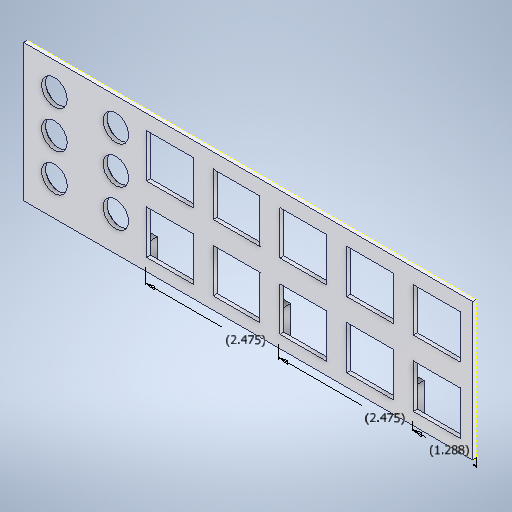
# Autodesk Inventor part: front_panel
Saved by Autodesk Inventor 2025 (Build 290162000, 162)
## iProperties
Created: 2025-05-12
Part Number: front_panel
Material: Generic
Document SubType Name: Modeling
Designer: ethan
Density: 1 g/cm^3
Appearance: PTFE
Author: ethan
Autodesk Inventor part; units mm, degrees
ref_plane "YZ Plane" through (0, 0, 0) normal (1, 0, 0) x (0, 1, 0)
ref_plane "XZ Plane" through (0, 0, 0) normal (0, 1, 0) x (-1, 0, 0)
ref_plane "XY Plane" through (0, 0, 0) normal (0, 0, 1) x (1, 0, 0)
sketch "Sketch1" plane through (0, 0, 0) normal (0, 0, 1) x (1, 0, 0)
  line L0 (0, 0) -> (-6.35, 0) construction
  line L1 (-6.35, 0) -> (-6.35, 6.35) construction
  line L2 (-6.35, 6.35) -> (0, 6.35) construction
  line L3 (0, 6.35) -> (0, 0) construction
  line L4 (-6.35, 6.35) -> (-30.1625, 6.35)
  line L5 (-30.1625, 6.35) -> (-30.1625, 28.575)
  line L6 (-30.1625, 28.575) -> (-6.35, 28.575)
  line L7 (-6.35, 28.575) -> (-6.35, 6.35)
  line L8 (-30.1625, 6.35) -> (-35.2425, 6.35) construction
  line L9 (-35.2425, 6.35) -> (-35.2425, 0) construction
  line L10 (-35.2425, 0) -> (-30.1625, 0) construction
  line L11 (-30.1625, 0) -> (-30.1625, 6.35) construction
  line L12 (-40.3225, 6.35) -> (-64.135, 6.35)
  line L13 (-64.135, 6.35) -> (-64.135, 28.575)
  line L14 (-64.135, 28.575) -> (-40.3225, 28.575)
  line L15 (-40.3225, 28.575) -> (-40.3225, 6.35)
  line L16 (-64.135, 6.35) -> (-69.215, 6.35) construction
  line L17 (-69.215, 6.35) -> (-69.215, 0) construction
  line L18 (-69.215, 0) -> (-64.135, 0) construction
  line L19 (-64.135, 0) -> (-64.135, 6.35) construction
  line L20 (-74.295, 6.35) -> (-98.1075, 6.35)
  line L21 (-98.1075, 6.35) -> (-98.1075, 28.575)
  line L22 (-98.1075, 28.575) -> (-74.295, 28.575)
  line L23 (-74.295, 28.575) -> (-74.295, 6.35)
  line L24 (-98.1075, 6.35) -> (-103.1875, 6.35) construction
  line L25 (-103.1875, 6.35) -> (-103.1875, 0) construction
  line L26 (-103.1875, 0) -> (-98.1075, 0) construction
  line L27 (-98.1075, 0) -> (-98.1075, 6.35) construction
  line L28 (-108.2675, 6.35) -> (-132.08, 6.35)
  line L29 (-132.08, 6.35) -> (-132.08, 28.575)
  line L30 (-132.08, 28.575) -> (-108.2675, 28.575)
  line L31 (-108.2675, 28.575) -> (-108.2675, 6.35)
  line L32 (-132.08, 6.35) -> (-137.16, 6.35) construction
  line L33 (-137.16, 6.35) -> (-137.16, 0) construction
  line L34 (-137.16, 0) -> (-132.08, 0) construction
  line L35 (-132.08, 0) -> (-132.08, 6.35) construction
  line L36 (-6.35, 40.005) -> (-30.1625, 40.005)
  line L37 (-30.1625, 40.005) -> (-30.1625, 62.23)
  line L38 (-30.1625, 62.23) -> (-6.35, 62.23)
  line L39 (-6.35, 62.23) -> (-6.35, 40.005)
  line L40 (-30.1625, 40.005) -> (-35.2425, 40.005) construction
  line L41 (-35.2425, 40.005) -> (-35.2425, 33.655) construction
  line L42 (-35.2425, 33.655) -> (-30.1625, 33.655) construction
  line L43 (-30.1625, 33.655) -> (-30.1625, 40.005) construction
  line L44 (-40.3225, 40.005) -> (-64.135, 40.005)
  line L45 (-64.135, 40.005) -> (-64.135, 62.23)
  line L46 (-64.135, 62.23) -> (-40.3225, 62.23)
  line L47 (-40.3225, 62.23) -> (-40.3225, 40.005)
  line L48 (-64.135, 40.005) -> (-69.215, 40.005) construction
  line L49 (-69.215, 40.005) -> (-69.215, 33.655) construction
  line L50 (-69.215, 33.655) -> (-64.135, 33.655) construction
  line L51 (-64.135, 33.655) -> (-64.135, 40.005) construction
  line L52 (-74.295, 40.005) -> (-98.1075, 40.005)
  line L53 (-98.1075, 40.005) -> (-98.1075, 62.23)
  line L54 (-98.1075, 62.23) -> (-74.295, 62.23)
  line L55 (-74.295, 62.23) -> (-74.295, 40.005)
  line L56 (-98.1075, 40.005) -> (-103.1875, 40.005) construction
  line L57 (-103.1875, 40.005) -> (-103.1875, 33.655) construction
  line L58 (-103.1875, 33.655) -> (-98.1075, 33.655) construction
  line L59 (-98.1075, 33.655) -> (-98.1075, 40.005) construction
  line L60 (-108.2675, 40.005) -> (-132.08, 40.005)
  line L61 (-132.08, 40.005) -> (-132.08, 62.23)
  line L62 (-132.08, 62.23) -> (-108.2675, 62.23)
  line L63 (-108.2675, 62.23) -> (-108.2675, 40.005)
  line L64 (-132.08, 40.005) -> (-137.16, 40.005) construction
  line L65 (-137.16, 40.005) -> (-137.16, 33.655) construction
  line L66 (-137.16, 33.655) -> (-132.08, 33.655) construction
  line L67 (-132.08, 33.655) -> (-132.08, 40.005) construction
  line L68 (0, -0.5542) -> (0, 69.2958)
  line L69 (0, 62.9458) -> (0, 69.2958)
  line L70 (-142.24, 6.35) -> (-166.0525, 6.35)
  line L71 (-166.0525, 6.35) -> (-166.0525, 28.575)
  line L72 (-166.0525, 28.575) -> (-142.24, 28.575)
  line L73 (-142.24, 28.575) -> (-142.24, 6.35)
  line L74 (-166.0525, 6.35) -> (-171.1325, 6.35) construction
  line L75 (-171.1325, 6.35) -> (-171.1325, 0) construction
  line L76 (-171.1325, 0) -> (-166.0525, 0) construction
  line L77 (-166.0525, 0) -> (-166.0525, 6.35) construction
  line L78 (-142.24, 40.005) -> (-166.0525, 40.005)
  line L79 (-166.0525, 40.005) -> (-166.0525, 62.23)
  line L80 (-166.0525, 62.23) -> (-142.24, 62.23)
  line L81 (-142.24, 62.23) -> (-142.24, 40.005)
  line L82 (-166.0525, 40.005) -> (-171.1325, 40.005) construction
  line L83 (-171.1325, 40.005) -> (-171.1325, 33.655) construction
  line L84 (-171.1325, 33.655) -> (-166.0525, 33.655) construction
  line L85 (-166.0525, 33.655) -> (-166.0525, 40.005) construction
  line L86 (0, 0) -> (-228.6, 0)
  line L87 (-228.6, 0) -> (-228.6, 69.85)
  line L88 (-228.6, 69.85) -> (0, 69.85)
  line L89 (0, 69.85) -> (0, 0)
  circle A0 centre (-181.6894, 55.6895) radius 6.5405
  line L90 (-228.6, 0) -> (-173.696, 0) construction
  line L91 (-173.696, 69.85) -> (-228.6, 69.85) construction
  line L92 (-228.6, 69.85) -> (-228.6, 0) construction
  line L93 (-228.6, 69.85) -> (-228.6, 42.1979) construction
  line L94 (-228.6, 42.1979) -> (-228.6, 34.925) construction
  line L95 (-228.6, 69.85) -> (-166.0525, 69.85) construction
  line L96 (-166.0525, 69.85) -> (-166.0525, 0) construction
  line L97 (-166.0525, 0) -> (-228.6, 0) construction
  line L98 (-228.6, 0) -> (-228.6, 69.85) construction
  line L99 (-166.0525, 69.85) -> (-197.3262, 69.85) construction
  line L100 (-197.3262, 69.85) -> (-197.3262, 0) construction
  line L101 (-197.3262, 0) -> (-166.0525, 0) construction
  line L102 (-166.0525, 0) -> (-166.0525, 69.85) construction
  circle A1 centre (-181.6894, 36.6395) radius 6.5405
  circle A2 centre (-181.6894, 17.5895) radius 6.5405
  circle A3 centre (-212.9631, 55.6895) radius 6.5405
  circle A4 centre (-212.9631, 36.6395) radius 6.5405
  circle A5 centre (-212.9631, 17.5895) radius 6.5405
  point P0 (-40.3225, 0)
  point P1 (-74.295, 0)
  point P2 (-108.2675, 0)
  point P3 (-6.35, 33.655)
  point P4 (-40.3225, 33.655)
  point P5 (-74.295, 33.655)
  point P6 (-108.2675, 33.655)
  point P7 (-142.24, 0)
  point P8 (-142.24, 33.655)
  point P9 (-181.6894, 69.85)
  dimension "d0" = 6.35
  dimension "d1" = 6.35
  dimension "d2" = 23.8125
  dimension "d3" = 22.225
  dimension "d4" = 5.08
  dimension "d7" = 33.9725
  dimension "d10" = 33.655
  dimension "d13" = 69.85
  dimension "d16" = 228.6
  dimension "d17" = 69.85
  dimension "d58" = 13.081
  dimension "d59" = 14.1605
  dimension "d62" = 19.05
  constraints: 206 end point, 13 parallel, 8 horizontal, 6 centre point, 6 perpendicular, 4 symmetric about line, 3 midpoint, 3 vertical, 2 coincident, 2 collinear, 2 point on line, 149 other
  measures "d0" distance of L1.end L2.end
  measures "d1" distance of L0.end L1.end
  measures "d2" distance of L5.end L6.end
  measures "d3" distance of L4.end L5.end
  measures "d4" distance of L10.end L9.end
  measures "d7" distance of L1.end L12.start
  measures "d10" distance of L1.end L36.start
  measures "d13" distance of L68.start L68.end
  measures "d16" distance of L87.end L88.end
  measures "d17" distance of L86.end L87.end
  measures "d58" diameter of A0
  measures "d59" distance of point (-181.689, 69.85) A0.centre
  measures "d62" distance of A0.centre A1.centre
extrude "Extrusion1" add sketch "Sketch1" along normal blind 2
sketch "Sketch3" plane through (0, 0, 0) normal (0, 0, -1) x (-1, 0, 0)
  line L0 (228.6, 69.85) -> (228.6, 0) projected
  line L1 (0, 69.85) -> (228.6, 69.85) projected
  line L2 (0, 0) -> (0, 69.85) projected
  line L3 (228.6, 0) -> (0, 0) projected
  circle A0 centre (181.6894, 55.6895) radius 6.5405 projected
  line L4 (142.24, 40.005) -> (166.0525, 40.005) projected
  line L5 (142.24, 62.23) -> (142.24, 40.005) projected
  line L6 (166.0525, 62.23) -> (142.24, 62.23) projected
  line L7 (166.0525, 40.005) -> (166.0525, 62.23) projected
  line L8 (142.24, 6.35) -> (166.0525, 6.35) projected
  line L9 (142.24, 28.575) -> (142.24, 6.35) projected
  line L10 (166.0525, 28.575) -> (142.24, 28.575) projected
  line L11 (166.0525, 6.35) -> (166.0525, 28.575) projected
  line L12 (108.2675, 40.005) -> (132.08, 40.005) projected
  line L13 (108.2675, 62.23) -> (108.2675, 40.005) projected
  line L14 (132.08, 62.23) -> (108.2675, 62.23) projected
  line L15 (132.08, 40.005) -> (132.08, 62.23) projected
  line L16 (74.295, 40.005) -> (98.1075, 40.005) projected
  line L17 (74.295, 62.23) -> (74.295, 40.005) projected
  line L18 (98.1075, 62.23) -> (74.295, 62.23) projected
  line L19 (98.1075, 40.005) -> (98.1075, 62.23) projected
  line L20 (40.3225, 40.005) -> (64.135, 40.005) projected
  line L21 (40.3225, 62.23) -> (40.3225, 40.005) projected
  line L22 (64.135, 62.23) -> (40.3225, 62.23) projected
  line L23 (64.135, 40.005) -> (64.135, 62.23) projected
  line L24 (6.35, 40.005) -> (30.1625, 40.005) projected
  line L25 (6.35, 62.23) -> (6.35, 40.005) projected
  line L26 (30.1625, 62.23) -> (6.35, 62.23) projected
  line L27 (30.1625, 40.005) -> (30.1625, 62.23) projected
  line L28 (108.2675, 6.35) -> (132.08, 6.35) projected
  line L29 (108.2675, 28.575) -> (108.2675, 6.35) projected
  line L30 (132.08, 28.575) -> (108.2675, 28.575) projected
  line L31 (132.08, 6.35) -> (132.08, 28.575) projected
  line L32 (74.295, 6.35) -> (98.1075, 6.35) projected
  line L33 (74.295, 28.575) -> (74.295, 6.35) projected
  line L34 (98.1075, 28.575) -> (74.295, 28.575) projected
  line L35 (98.1075, 6.35) -> (98.1075, 28.575) projected
  line L36 (40.3225, 6.35) -> (64.135, 6.35) projected
  line L37 (40.3225, 28.575) -> (40.3225, 6.35) projected
  line L38 (64.135, 28.575) -> (40.3225, 28.575) projected
  line L39 (64.135, 6.35) -> (64.135, 28.575) projected
  line L40 (6.35, 6.35) -> (30.1625, 6.35) projected
  line L41 (6.35, 28.575) -> (6.35, 6.35) projected
  line L42 (30.1625, 28.575) -> (6.35, 28.575) projected
  line L43 (30.1625, 6.35) -> (30.1625, 28.575) projected
  line L44 (3.81, 37.465) -> (32.7025, 37.465)
  line L45 (32.7025, 37.465) -> (32.7025, 64.77)
  line L46 (32.7025, 64.77) -> (3.81, 64.77)
  line L47 (3.81, 64.77) -> (3.81, 37.465)
  line L48 (37.7825, 37.465) -> (66.675, 37.465)
  line L49 (66.675, 37.465) -> (66.675, 64.77)
  line L50 (66.675, 64.77) -> (37.7825, 64.77)
  line L51 (37.7825, 64.77) -> (37.7825, 37.465)
  line L52 (71.755, 37.465) -> (100.6475, 37.465)
  line L53 (100.6475, 37.465) -> (100.6475, 64.77)
  line L54 (100.6475, 64.77) -> (71.755, 64.77)
  line L55 (71.755, 64.77) -> (71.755, 37.465)
  line L56 (105.7275, 37.465) -> (134.62, 37.465)
  line L57 (134.62, 37.465) -> (134.62, 64.77)
  line L58 (134.62, 64.77) -> (105.7275, 64.77)
  line L59 (105.7275, 64.77) -> (105.7275, 37.465)
  line L60 (139.7, 37.465) -> (168.5925, 37.465)
  line L61 (168.5925, 37.465) -> (168.5925, 64.77)
  line L62 (168.5925, 64.77) -> (139.7, 64.77)
  line L63 (139.7, 64.77) -> (139.7, 37.465)
  line L64 (139.7, 3.81) -> (168.5925, 3.81)
  line L65 (168.5925, 3.81) -> (168.5925, 31.115)
  line L66 (168.5925, 31.115) -> (139.7, 31.115)
  line L67 (139.7, 31.115) -> (139.7, 3.81)
  line L68 (105.7275, 3.81) -> (134.62, 3.81)
  line L69 (134.62, 3.81) -> (134.62, 31.115)
  line L70 (134.62, 31.115) -> (105.7275, 31.115)
  line L71 (105.7275, 31.115) -> (105.7275, 3.81)
  line L72 (71.755, 3.81) -> (100.6475, 3.81)
  line L73 (100.6475, 3.81) -> (100.6475, 31.115)
  line L74 (100.6475, 31.115) -> (71.755, 31.115)
  line L75 (71.755, 31.115) -> (71.755, 3.81)
  line L76 (37.7825, 3.81) -> (66.675, 3.81)
  line L77 (66.675, 3.81) -> (66.675, 31.115)
  line L78 (66.675, 31.115) -> (37.7825, 31.115)
  line L79 (37.7825, 31.115) -> (37.7825, 3.81)
  line L80 (3.81, 3.81) -> (32.7025, 3.81)
  line L81 (32.7025, 3.81) -> (32.7025, 31.115)
  line L82 (32.7025, 31.115) -> (3.81, 31.115)
  line L83 (3.81, 31.115) -> (3.81, 3.81)
  line L84 (228.6, 69.85) -> (228.6, 0) projected
  line L85 (0, 69.85) -> (228.6, 69.85) projected
  line L86 (0, 0) -> (0, 69.85) projected
  line L87 (228.6, 0) -> (0, 0) projected
  circle A1 centre (181.6894, 55.6895) radius 6.5405 projected
  circle A2 centre (181.6894, 36.6395) radius 6.5405 projected
  circle A3 centre (181.6894, 17.5895) radius 6.5405 projected
  circle A4 centre (212.9631, 36.6395) radius 6.5405 projected
  circle A5 centre (212.9631, 55.6895) radius 6.5405 projected
  circle A6 centre (212.9631, 17.5895) radius 6.5405 projected
  line L88 (142.24, 40.005) -> (166.0525, 40.005) projected
  line L89 (142.24, 62.23) -> (142.24, 40.005) projected
  line L90 (166.0525, 62.23) -> (142.24, 62.23) projected
  line L91 (166.0525, 40.005) -> (166.0525, 62.23) projected
  line L92 (142.24, 6.35) -> (166.0525, 6.35) projected
  line L93 (142.24, 28.575) -> (142.24, 6.35) projected
  line L94 (166.0525, 28.575) -> (142.24, 28.575) projected
  line L95 (166.0525, 6.35) -> (166.0525, 28.575) projected
  line L96 (108.2675, 40.005) -> (132.08, 40.005) projected
  line L97 (108.2675, 62.23) -> (108.2675, 40.005) projected
  line L98 (132.08, 62.23) -> (108.2675, 62.23) projected
  line L99 (132.08, 40.005) -> (132.08, 62.23) projected
  line L100 (74.295, 40.005) -> (98.1075, 40.005) projected
  line L101 (74.295, 62.23) -> (74.295, 40.005) projected
  line L102 (98.1075, 62.23) -> (74.295, 62.23) projected
  line L103 (98.1075, 40.005) -> (98.1075, 62.23) projected
  line L104 (40.3225, 40.005) -> (64.135, 40.005) projected
  line L105 (40.3225, 62.23) -> (40.3225, 40.005) projected
  line L106 (64.135, 62.23) -> (40.3225, 62.23) projected
  line L107 (64.135, 40.005) -> (64.135, 62.23) projected
  line L108 (6.35, 40.005) -> (30.1625, 40.005) projected
  line L109 (6.35, 62.23) -> (6.35, 40.005) projected
  line L110 (30.1625, 62.23) -> (6.35, 62.23) projected
  line L111 (30.1625, 40.005) -> (30.1625, 62.23) projected
  line L112 (108.2675, 6.35) -> (132.08, 6.35) projected
  line L113 (108.2675, 28.575) -> (108.2675, 6.35) projected
  line L114 (132.08, 28.575) -> (108.2675, 28.575) projected
  line L115 (132.08, 6.35) -> (132.08, 28.575) projected
  line L116 (74.295, 6.35) -> (98.1075, 6.35) projected
  line L117 (74.295, 28.575) -> (74.295, 6.35) projected
  line L118 (98.1075, 28.575) -> (74.295, 28.575) projected
  line L119 (98.1075, 6.35) -> (98.1075, 28.575) projected
  line L120 (40.3225, 6.35) -> (64.135, 6.35) projected
  line L121 (40.3225, 28.575) -> (40.3225, 6.35) projected
  line L122 (64.135, 28.575) -> (40.3225, 28.575) projected
  line L123 (64.135, 6.35) -> (64.135, 28.575) projected
  line L124 (6.35, 6.35) -> (30.1625, 6.35) projected
  line L125 (6.35, 28.575) -> (6.35, 6.35) projected
  line L126 (30.1625, 28.575) -> (6.35, 28.575) projected
  line L127 (30.1625, 6.35) -> (30.1625, 28.575) projected
  circle A7 centre (181.6894, 55.6895) radius 9.0805
  circle A8 centre (212.9631, 55.6895) radius 9.0805
  circle A9 centre (212.9631, 36.6395) radius 9.0805
  circle A10 centre (212.9631, 17.5895) radius 9.0805
  circle A11 centre (181.6894, 17.5895) radius 9.0805
  circle A12 centre (181.6894, 36.6395) radius 9.0805
  dimension "d48" = 2.54
  dimension "d49" = 2.54
  dimension "d50" = 2.54
  dimension "d51" = 2.54
  dimension "d52" = 2.54
  dimension "d53" = 2.54
  dimension "d54" = 2.54
  dimension "d55" = 2.54
  dimension "d56" = 2.54
  dimension "d57" = 2.54
  dimension "d67" = 2.54
  dimension "d68" = 2.54
  dimension "d69" = 2.54
  dimension "d70" = 2.54
  dimension "d71" = 2.54
  dimension "d72" = 2.54
  constraints: 80 end point, 6 centre point, 30 other
  measures "d48" distance between parallel lines of L25 L47
  measures "d49" distance between parallel lines of L21 L51
  measures "d50" distance between parallel lines of L17 L55
  measures "d51" distance between parallel lines of L13 L59
  measures "d52" distance between parallel lines of L5 L63
  measures "d53" distance between parallel lines of L9 L67
  measures "d54" distance between parallel lines of L29 L71
  measures "d55" distance between parallel lines of L33 L75
  measures "d56" distance between parallel lines of L37 L79
  measures "d57" distance between parallel lines of L41 L83
  measures "d67" radial gap between concentric circles of A0 A7
  measures "d68" radial gap between concentric circles of A5 A8
  measures "d69" radial gap between concentric circles of A4 A9
  measures "d70" radial gap between concentric circles of A6 A10
  measures "d71" radial gap between concentric circles of A3 A11
  measures "d72" radial gap between concentric circles of A2 A12
extrude "Extrusion2" add sketch "Sketch3" along normal blind 2 contours L0 L3 L2 L1
sketch "Sketch4" plane through (0, 0, -2) normal (0, 0, -1) x (-1, 0, 0)
  line L0 (228.6, 0) -> (228.6, 69.85) construction
  line L1 (228.6, 69.85) -> (0, 69.85) construction
  line L2 (0, 69.85) -> (0, 0) construction
  line L3 (0, 0) -> (228.6, 0) construction
  circle A0 centre (181.6894, 36.6395) radius 9.0805 construction
  circle A1 centre (181.6894, 17.5895) radius 9.0805 construction
  circle A2 centre (212.9631, 17.5895) radius 9.0805 construction
  circle A3 centre (212.9631, 36.6395) radius 9.0805 construction
  circle A4 centre (212.9631, 55.6895) radius 9.0805 construction
  circle A5 centre (181.6894, 55.6895) radius 9.0805 construction
  line L4 (3.81, 3.81) -> (3.81, 31.115) construction
  line L5 (3.81, 31.115) -> (32.7025, 31.115) construction
  line L6 (32.7025, 31.115) -> (32.7025, 3.81) construction
  line L7 (32.7025, 3.81) -> (3.81, 3.81) construction
  line L8 (37.7825, 3.81) -> (37.7825, 31.115) construction
  line L9 (37.7825, 31.115) -> (66.675, 31.115) construction
  line L10 (66.675, 31.115) -> (66.675, 3.81) construction
  line L11 (66.675, 3.81) -> (37.7825, 3.81) construction
  line L12 (71.755, 3.81) -> (71.755, 31.115) construction
  line L13 (71.755, 31.115) -> (100.6475, 31.115) construction
  line L14 (100.6475, 31.115) -> (100.6475, 3.81) construction
  line L15 (100.6475, 3.81) -> (71.755, 3.81) construction
  line L16 (105.7275, 3.81) -> (105.7275, 31.115) construction
  line L17 (105.7275, 31.115) -> (134.62, 31.115) construction
  line L18 (134.62, 31.115) -> (134.62, 3.81) construction
  line L19 (134.62, 3.81) -> (105.7275, 3.81) construction
  line L20 (139.7, 3.81) -> (139.7, 31.115) construction
  line L21 (139.7, 31.115) -> (168.5925, 31.115) construction
  line L22 (168.5925, 31.115) -> (168.5925, 3.81) construction
  line L23 (168.5925, 3.81) -> (139.7, 3.81) construction
  line L24 (139.7, 37.465) -> (139.7, 64.77) construction
  line L25 (139.7, 64.77) -> (168.5925, 64.77) construction
  line L26 (168.5925, 64.77) -> (168.5925, 37.465) construction
  line L27 (168.5925, 37.465) -> (139.7, 37.465) construction
  line L28 (105.7275, 37.465) -> (105.7275, 64.77) construction
  line L29 (105.7275, 64.77) -> (134.62, 64.77) construction
  line L30 (134.62, 64.77) -> (134.62, 37.465) construction
  line L31 (134.62, 37.465) -> (105.7275, 37.465) construction
  line L32 (71.755, 37.465) -> (71.755, 64.77) construction
  line L33 (71.755, 64.77) -> (100.6475, 64.77) construction
  line L34 (100.6475, 64.77) -> (100.6475, 37.465) construction
  line L35 (100.6475, 37.465) -> (71.755, 37.465) construction
  line L36 (37.7825, 37.465) -> (37.7825, 64.77) construction
  line L37 (37.7825, 64.77) -> (66.675, 64.77) construction
  line L38 (66.675, 64.77) -> (66.675, 37.465) construction
  line L39 (66.675, 37.465) -> (37.7825, 37.465) construction
  line L40 (3.81, 37.465) -> (3.81, 64.77) construction
  line L41 (3.81, 64.77) -> (32.7025, 64.77) construction
  line L42 (32.7025, 64.77) -> (32.7025, 37.465) construction
  line L43 (32.7025, 37.465) -> (3.81, 37.465) construction
  line L44 (0, 69.85) -> (2, 69.85)
  line L45 (2, 69.85) -> (2, 0)
  line L46 (2, 0) -> (0, 0)
  line L47 (0, 0) -> (0, 69.85)
  line L48 (228.6, 69.85) -> (226.6, 69.85)
  line L49 (226.6, 69.85) -> (226.6, 0)
  line L50 (226.6, 0) -> (228.6, 0)
  line L51 (228.6, 0) -> (228.6, 69.85)
  dimension "d75" = 2
  dimension "d76" = 2
  constraints: 16 end point, 4 parallel, 2 horizontal, 2 perpendicular, 2 point on line
  measures "d75" distance of L45.end L46.end
  measures "d76" distance of L50.end L49.end
extrude "Extrusion3" cut sketch "Sketch4" against normal blind 2
sketch "Sketch5" plane through (0, 0, -2) normal (0, 0, -1) x (-1, 0, 0)
  line L0 (2, 0) -> (226.6, 0) projected
  line L1 (226.6, 0) -> (226.6, 69.85) projected
  line L2 (2, 0) -> (226.6, 0)
  line L3 (226.6, 0) -> (226.6, 2)
  line L4 (226.6, 2) -> (2, 2)
  line L5 (2, 2) -> (2, 0)
  line L6 (2, 69.85) -> (2, 0) construction
  line L7 (2, 0) -> (226.6, 0) construction
  line L8 (226.6, 0) -> (226.6, 69.85) construction
  line L9 (226.6, 69.85) -> (2, 69.85) construction
  circle A0 centre (181.6894, 36.6395) radius 9.0805 construction
  circle A1 centre (181.6894, 17.5895) radius 9.0805 construction
  circle A2 centre (212.9631, 17.5895) radius 9.0805 construction
  circle A3 centre (212.9631, 36.6395) radius 9.0805 construction
  circle A4 centre (212.9631, 55.6895) radius 9.0805 construction
  circle A5 centre (181.6894, 55.6895) radius 9.0805 construction
  line L10 (3.81, 3.81) -> (3.81, 31.115) construction
  line L11 (3.81, 31.115) -> (32.7025, 31.115) construction
  line L12 (32.7025, 31.115) -> (32.7025, 3.81) construction
  line L13 (32.7025, 3.81) -> (3.81, 3.81) construction
  line L14 (37.7825, 3.81) -> (37.7825, 31.115) construction
  line L15 (37.7825, 31.115) -> (66.675, 31.115) construction
  line L16 (66.675, 31.115) -> (66.675, 3.81) construction
  line L17 (66.675, 3.81) -> (37.7825, 3.81) construction
  line L18 (71.755, 3.81) -> (71.755, 31.115) construction
  line L19 (71.755, 31.115) -> (100.6475, 31.115) construction
  line L20 (100.6475, 31.115) -> (100.6475, 3.81) construction
  line L21 (100.6475, 3.81) -> (71.755, 3.81) construction
  line L22 (105.7275, 3.81) -> (105.7275, 31.115) construction
  line L23 (105.7275, 31.115) -> (134.62, 31.115) construction
  line L24 (134.62, 31.115) -> (134.62, 3.81) construction
  line L25 (134.62, 3.81) -> (105.7275, 3.81) construction
  line L26 (139.7, 3.81) -> (139.7, 31.115) construction
  line L27 (139.7, 31.115) -> (168.5925, 31.115) construction
  line L28 (168.5925, 31.115) -> (168.5925, 3.81) construction
  line L29 (168.5925, 3.81) -> (139.7, 3.81) construction
  line L30 (139.7, 37.465) -> (139.7, 64.77) construction
  line L31 (139.7, 64.77) -> (168.5925, 64.77) construction
  line L32 (168.5925, 64.77) -> (168.5925, 37.465) construction
  line L33 (168.5925, 37.465) -> (139.7, 37.465) construction
  line L34 (105.7275, 37.465) -> (105.7275, 64.77) construction
  line L35 (105.7275, 64.77) -> (134.62, 64.77) construction
  line L36 (134.62, 64.77) -> (134.62, 37.465) construction
  line L37 (134.62, 37.465) -> (105.7275, 37.465) construction
  line L38 (71.755, 37.465) -> (71.755, 64.77) construction
  line L39 (71.755, 64.77) -> (100.6475, 64.77) construction
  line L40 (100.6475, 64.77) -> (100.6475, 37.465) construction
  line L41 (100.6475, 37.465) -> (71.755, 37.465) construction
  line L42 (37.7825, 37.465) -> (37.7825, 64.77) construction
  line L43 (37.7825, 64.77) -> (66.675, 64.77) construction
  line L44 (66.675, 64.77) -> (66.675, 37.465) construction
  line L45 (66.675, 37.465) -> (37.7825, 37.465) construction
  line L46 (3.81, 37.465) -> (3.81, 64.77) construction
  line L47 (3.81, 64.77) -> (32.7025, 64.77) construction
  line L48 (32.7025, 64.77) -> (32.7025, 37.465) construction
  line L49 (32.7025, 37.465) -> (3.81, 37.465) construction
  line L50 (2, 69.85) -> (226.6, 69.85) construction
  line L51 (226.6, 69.85) -> (226.6, 67.85) construction
  line L52 (226.6, 67.85) -> (2, 67.85) construction
  line L53 (2, 67.85) -> (2, 69.85) construction
  line L54 (2, 67.85) -> (226.6, 67.85)
  line L55 (226.6, 67.85) -> (226.6, 69.85)
  line L56 (226.6, 69.85) -> (2, 69.85)
  line L57 (2, 69.85) -> (2, 67.85)
  point P0 (0, 0)
  dimension "d79" = 2
  dimension "d80" = 2
  constraints: 24 end point, 6 parallel, 3 horizontal, 3 perpendicular, 2 point on line
  measures "d79" distance of L3.end L2.end
  measures "d80" distance of L50.end L51.end
extrude "Extrusion4" cut sketch "Sketch5" against normal blind 2
sketch "Sketch6" plane through (0, 0, -2) normal (0, 0, -1) x (-1, 0, 0)
  line L0 (2, 2) -> (226.6, 2) construction
  line L1 (226.6, 2) -> (226.6, 67.85) construction
  line L2 (226.6, 67.85) -> (2, 67.85) construction
  line L3 (2, 67.85) -> (2, 2) construction
  circle A0 centre (181.6894, 36.6395) radius 9.0805 construction
  circle A1 centre (181.6894, 17.5895) radius 9.0805 construction
  circle A2 centre (212.9631, 17.5895) radius 9.0805 construction
  circle A3 centre (212.9631, 36.6395) radius 9.0805 construction
  circle A4 centre (212.9631, 55.6895) radius 9.0805 construction
  circle A5 centre (181.6894, 55.6895) radius 9.0805 construction
  line L4 (3.81, 3.81) -> (3.81, 31.115) construction
  line L5 (3.81, 31.115) -> (32.7025, 31.115) construction
  line L6 (32.7025, 31.115) -> (32.7025, 3.81) construction
  line L7 (32.7025, 3.81) -> (3.81, 3.81) construction
  line L8 (37.7825, 3.81) -> (37.7825, 31.115) construction
  line L9 (37.7825, 31.115) -> (66.675, 31.115) construction
  line L10 (66.675, 31.115) -> (66.675, 3.81) construction
  line L11 (66.675, 3.81) -> (37.7825, 3.81) construction
  line L12 (71.755, 3.81) -> (71.755, 31.115) construction
  line L13 (71.755, 31.115) -> (100.6475, 31.115) construction
  line L14 (100.6475, 31.115) -> (100.6475, 3.81) construction
  line L15 (100.6475, 3.81) -> (71.755, 3.81) construction
  line L16 (105.7275, 3.81) -> (105.7275, 31.115) construction
  line L17 (105.7275, 31.115) -> (134.62, 31.115) construction
  line L18 (134.62, 31.115) -> (134.62, 3.81) construction
  line L19 (134.62, 3.81) -> (105.7275, 3.81) construction
  line L20 (139.7, 3.81) -> (139.7, 31.115) construction
  line L21 (139.7, 31.115) -> (168.5925, 31.115) construction
  line L22 (168.5925, 31.115) -> (168.5925, 3.81) construction
  line L23 (168.5925, 3.81) -> (139.7, 3.81) construction
  line L24 (139.7, 37.465) -> (139.7, 64.77) construction
  line L25 (139.7, 64.77) -> (168.5925, 64.77) construction
  line L26 (168.5925, 64.77) -> (168.5925, 37.465) construction
  line L27 (168.5925, 37.465) -> (139.7, 37.465) construction
  line L28 (105.7275, 37.465) -> (105.7275, 64.77) construction
  line L29 (105.7275, 64.77) -> (134.62, 64.77) construction
  line L30 (134.62, 64.77) -> (134.62, 37.465) construction
  line L31 (134.62, 37.465) -> (105.7275, 37.465) construction
  line L32 (71.755, 37.465) -> (71.755, 64.77) construction
  line L33 (71.755, 64.77) -> (100.6475, 64.77) construction
  line L34 (100.6475, 64.77) -> (100.6475, 37.465) construction
  line L35 (100.6475, 37.465) -> (71.755, 37.465) construction
  line L36 (37.7825, 37.465) -> (37.7825, 64.77) construction
  line L37 (37.7825, 64.77) -> (66.675, 64.77) construction
  line L38 (66.675, 64.77) -> (66.675, 37.465) construction
  line L39 (66.675, 37.465) -> (37.7825, 37.465) construction
  line L40 (3.81, 37.465) -> (3.81, 64.77) construction
  line L41 (3.81, 64.77) -> (32.7025, 64.77) construction
  line L42 (32.7025, 64.77) -> (32.7025, 37.465) construction
  line L43 (32.7025, 37.465) -> (3.81, 37.465) construction
  line L44 (37.7825, 3.81) -> (37.7825, 31.115) construction
  line L45 (32.7025, 2) -> (37.7825, 2) construction
  line L46 (37.7825, 2) -> (37.7825, 14.7) construction
  line L47 (37.7825, 14.7) -> (32.7025, 14.7) construction
  line L48 (32.7025, 14.7) -> (32.7025, 2) construction
  line L49 (228.6, 0) -> (0, 0) construction
  line L50 (228.6, 69.85) -> (228.6, 0) construction
  line L51 (0, 69.85) -> (228.6, 69.85) construction
  line L52 (0, 0) -> (0, 69.85) construction
  line L53 (2, 2) -> (226.6, 2) construction
  line L54 (2, 67.85) -> (2, 2) construction
  line L55 (226.6, 67.85) -> (2, 67.85) construction
  line L56 (226.6, 2) -> (226.6, 67.85) construction
  line L57 (32.7025, 0) -> (37.7825, 0) construction
  line L58 (37.7825, 0) -> (37.7825, 10.16) construction
  line L59 (37.7825, 10.16) -> (32.7025, 10.16) construction
  line L60 (32.7025, 10.16) -> (32.7025, 0) construction
  line L61 (32.7025, 0) -> (37.7825, 0) construction
  line L62 (37.7825, 0) -> (37.7825, 14.7) construction
  line L63 (37.7825, 14.7) -> (32.7025, 14.7) construction
  line L64 (32.7025, 14.7) -> (32.7025, 0) construction
  line L65 (37.7825, 14.7) -> (32.7025, 14.7)
  line L66 (32.7025, 14.7) -> (32.7025, 0)
  line L67 (32.7025, 0) -> (37.7825, 0)
  line L68 (37.7825, 0) -> (37.7825, 14.7)
  line L69 (105.7275, 14.7) -> (100.6475, 14.7)
  line L70 (100.6475, 14.7) -> (100.6475, 0)
  line L71 (100.6475, 0) -> (105.7275, 0)
  line L72 (105.7275, 0) -> (105.7275, 14.7)
  line L73 (168.5925, 0) -> (173.6725, 0)
  line L74 (173.6725, 0) -> (173.6725, 10.16)
  line L75 (173.6725, 10.16) -> (168.5925, 10.16)
  line L76 (168.5925, 10.16) -> (168.5925, 0)
  dimension "d83" = 12.7
  dimension "d84" = 10.16
  dimension "d85" = 5.08
  dimension "d86" = 10.16
  constraints: 48 end point, 12 parallel, 7 point on line, 6 horizontal, 6 perpendicular
  measures "d83" distance of L46.end L45.end
  measures "d84" distance of L58.end L57.end
  measures "d85" distance of L75.end L74.end
  measures "d86" distance of L74.end L73.end
extrude "Extrusion5" add sketch "Sketch6" along normal blind 4 and the other way blind 2
sketch "Sketch7" plane through (0, 0, 0) normal (0, 0, -1) x (-1, 0, 0)
  line L0 (173.6725, 2) -> (173.6725, 0) construction
  line L1 (228.6, 0) -> (173.6725, 0) construction
  line L2 (228.6, 69.85) -> (228.6, 0) construction
  line L3 (0, 69.85) -> (228.6, 69.85) construction
  line L4 (0, 0) -> (0, 69.85) construction
  line L5 (32.7025, 0) -> (0, 0) construction
  line L6 (32.7025, 0) -> (32.7025, 2) construction
  line L7 (2, 2) -> (32.7025, 2) construction
  line L8 (2, 67.85) -> (2, 2) construction
  line L9 (226.6, 67.85) -> (2, 67.85) construction
  line L10 (226.6, 2) -> (226.6, 67.85) construction
  line L11 (173.6725, 2) -> (226.6, 2) construction
  line L12 (100.6475, 0) -> (100.6475, 2) construction
  line L13 (37.7825, 2) -> (100.6475, 2) construction
  line L14 (37.7825, 2) -> (37.7825, 0) construction
  line L15 (100.6475, 0) -> (37.7825, 0) construction
  line L16 (168.5925, 0) -> (168.5925, 2) construction
  line L17 (105.7275, 2) -> (168.5925, 2) construction
  line L18 (105.7275, 2) -> (105.7275, 0) construction
  line L19 (168.5925, 0) -> (105.7275, 0) construction
  line L20 (32.7025, 14.7) -> (32.7025, 0) construction
  line L21 (32.7025, 0) -> (37.7825, 0) construction
  line L22 (37.7825, 0) -> (37.7825, 14.7) construction
  line L23 (37.7825, 14.7) -> (32.7025, 14.7) construction
  line L24 (100.6475, 14.7) -> (100.6475, 0) construction
  line L25 (100.6475, 0) -> (105.7275, 0) construction
  line L26 (105.7275, 0) -> (105.7275, 14.7) construction
  line L27 (105.7275, 14.7) -> (100.6475, 14.7) construction
  line L28 (173.6725, 0) -> (173.6725, 10.16) construction
  line L29 (173.6725, 10.16) -> (168.5925, 10.16) construction
  line L30 (168.5925, 10.16) -> (168.5925, 0) construction
  line L31 (168.5925, 0) -> (173.6725, 0) construction
  line L32 (0, 0) -> (32.7025, 0) construction
  dimension "d91" = 32.7025
  dimension "d92" = 62.865
  dimension "d93" = 62.865
  constraints: 2 end point, 1 collinear
  measures "d91" distance of L5.start L4.start
  measures "d92" distance of L12.start L14.end
  measures "d93" distance of L16.start L18.end
body "Solid1"
